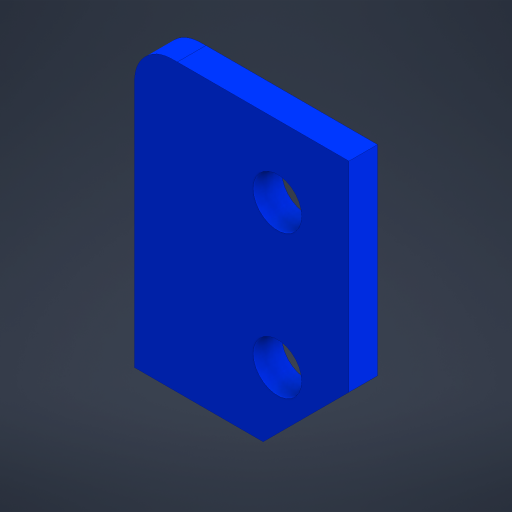
# Autodesk Inventor part: Belt Holders
Saved by Autodesk Inventor 2024.2 (Build 282272000, 272)
## iProperties
Created: 2024-10-17
Part Number: Belt Holders
Material: Generic
Document SubType Name: Modeling
Designer: jerem
Density: 1 g/cm^3
Appearance: Default
Author: jerem
Autodesk Inventor part; units mm, degrees
ref_plane "YZ Plane" through (0, 0, 0) normal (1, 0, 0) x (0, 1, 0)
ref_plane "XZ Plane" through (0, 0, 0) normal (0, 1, 0) x (-1, 0, 0)
ref_plane "XY Plane" through (0, 0, 0) normal (0, 0, 1) x (1, 0, 0)
sketch "Sketch1" plane through (0, 0, 0) normal (0, 0, 1) x (1, 0, 0)
  line L0 (0, 0) -> (15, 0)
  line L1 (15, 0) -> (15, 20)
  line L2 (15, 20) -> (0, 20)
  line L3 (0, 20) -> (0, 0)
  circle A0 centre (10, 15) radius 1.7
  circle A1 centre (10, 5) radius 1.7
  line L4 (10, 15) -> (10, 0) construction
  dimension "d0" = 15
  dimension "d1" = 20
  dimension "d2" = 3.4
  dimension "d3" = 3.4
  dimension "d5" = 15
  dimension "d6" = 5
  dimension "d7" = 5
  constraints: 10 end point, 2 centre point, 2 parallel, 2 perpendicular, 2 point on line, 1 horizontal
  measures "d0" distance of L1.end L2.end
  measures "d1" distance of L0.end L1.end
  measures "d2" diameter of A0
  measures "d3" diameter of A1
  measures "d5" distance of L4.end L4.start
  measures "d6" distance of L4.end A1.centre
  measures "d7" distance between parallel lines of L1 L4
extrude "Extrusion1" add sketch "Sketch1" along normal blind 2
chamfer "Chamfer1" distance 6 angle 45 1 edges at (15, 0, 1)
fillet "Fillet1" radius 3 1 edges at (0, 20, 1) curvature continuous yes
equation "\"d3\" = d2"
body "Solid1"
